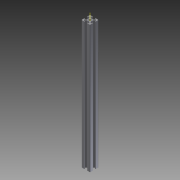
# Autodesk Inventor part: profile
Saved by Autodesk Inventor 2012 (Build 160160000, 160)
## iProperties
Created: 2013-02-18
Part Number: profile
Material: Default
Document SubType Name: Modeling
Designer: mce
Density: 1 g/cm^3
Mass: 59.1534 g
Surface Area: 620.774 cm^2
Volume: 59.1534 cm^3
Author: mce
Autodesk Inventor part; units mm, degrees
ref_plane "YZ Plane" through (0, 0, 0) normal (1, 0, 0) x (0, 1, 0)
ref_plane "XZ Plane" through (0, 0, 0) normal (0, 1, 0) x (-1, 0, 0)
ref_plane "XY Plane" through (0, 0, 0) normal (0, 0, 1) x (1, 0, 0)
sketch "Sketch1" plane through (0, 0, 0) normal (0, 0, 1) x (1, 0, 0)
  line L0 (6.4, 0) -> (1.2, 0)
  line L1 (0, 1.2) -> (0, 6.4)
  line L2 (0.5, 6.9) -> (1.4, 6.9)
  line L3 (1.4, 6.9) -> (1.4, 3.9)
  line L4 (2.4858, 3.9) -> (5.7, 7.1142)
  line L5 (5.7, 7.1142) -> (5.7, 9.8)
  line L6 (3.9, 2.4858) -> (7.1142, 5.7)
  line L7 (7.1142, 5.7) -> (9.8, 5.7)
  line L8 (7.1435, 8.5577) -> (7.6727, 9.0869)
  line L9 (8.5577, 7.1435) -> (9.0869, 7.6727)
  line L10 (6.9, 0.5) -> (6.9, 1.4)
  line L11 (6.9, 1.4) -> (3.9, 1.4)
  line L12 (5.9, 10) -> (24.7723, 10) construction
  line L13 (10, 21.5486) -> (10, 5.9) construction
  line L14 (1.4, 3.9) -> (2.4858, 3.9)
  line L15 (3.9, 1.4) -> (3.9, 2.4858)
  arc A0 (7.5, 10) -> (7.6727, 9.0869) centre (10, 10) ccw
  arc A1 (9.0869, 7.6727) -> (10, 7.5) centre (10, 10) ccw
  line L16 (14.358, 14.358) -> (-3.5262, -3.5262) construction
  arc A2 (7.1435, 8.5577) -> (8.5577, 7.1435) centre (10, 10) ccw
  line L17 (7.5, 10) -> (5.9, 10)
  line L18 (10, 7.5) -> (10, 5.9)
  arc A3 (0, 1.2) -> (1.2, 0) centre (1.2, 1.2) ccw
  line L19 (0, 6.4) -> (0.5, 6.9)
  line L20 (6.4, 0) -> (6.9, 0.5)
  line L21 (5.7, 9.8) -> (5.9, 10)
  line L22 (10, 5.9) -> (9.8, 5.7)
  point P0 (0, 0)
  point P1 (6.9, 0)
  point P2 (0, 6.9)
  point P3 (5.7, 10)
  point P4 (10, 5.7)
  dimension "d0" = 10
  dimension "d1" = 10
  dimension "d3" = 1.4
  dimension "d4" = 6.1
  dimension "d5" = 6.1
  dimension "d6" = 3.1
  dimension "d7" = 3.1
  dimension "d9" = 5.7
  dimension "d10" = 5.7
  dimension "d12" = 2
  dimension "d14" = 2.5
  dimension "d15" = 3.2
  dimension "d21" = 1.2
  dimension "d22" = 0.5
  dimension "d23" = 0.5
  dimension "d24" = 0.5
  dimension "d25" = 0.5
  dimension "d26" = 0.2
  dimension "d27" = 0.2
  dimension "d28" = 0.2
  dimension "d29" = 0.2
  constraints: 46 end point, 14 point on line, 8 point on circle, 7 perpendicular, 6 parallel, 4 centre point, 4 collinear, 3 tangent, 1 coincident, 1 horizontal, 1 horizontal alignment, 1 vertical alignment, 1 other
  measures "d0" distance between parallel lines of L13 L1
  measures "d1" distance between parallel lines of L12 L0
  measures "d3" distance between parallel lines of L11 L0
  measures "d4" distance between parallel lines of L12 L14
  measures "d5" distance between parallel lines of L13 L15
  measures "d6" distance between parallel lines of L12 L2
  measures "d7" distance between parallel lines of L13 L10
  measures "d9" distance between parallel lines of L1 L5
  measures "d10" distance between parallel lines of L0 L7
  measures "d12" distance between parallel lines of L6 L4
  measures "d14" radius of A0
  measures "d15" radius of A2
  measures "d21" radius of A3
  measures "d22" distance of L1.end point (0, 6.9)
  measures "d23" distance of L2.start point (0, 6.9)
  measures "d24" distance of L0.start point (6.9, 0)
  measures "d25" distance of L10.start point (6.9, 0)
  measures "d26" distance of L5.end point (5.7, 10)
  measures "d27" distance of L12.start point (5.7, 10)
  measures "d28" distance of L13.end point (10, 5.7)
  measures "d29" distance of L7.end point (10, 5.7)
extrude "Extrusion2" add sketch "Sketch1" along normal blind 300
pattern_circular "Circular Pattern2" count 4 over 360 about axis through (10, 10, 300) along (0, 0, 1) of "Extrusion2"
equation "\"d5\" = d4"
equation "\"d7\" = d6"
equation "\"d10\" = d9"
equation "\"d23\" = d22"
equation "\"d24\" = d22"
equation "\"d25\" = d24"
equation "\"d27\" = d26"
equation "\"d28\" = d26"
equation "\"d29\" = d28"
body "Solid2"
